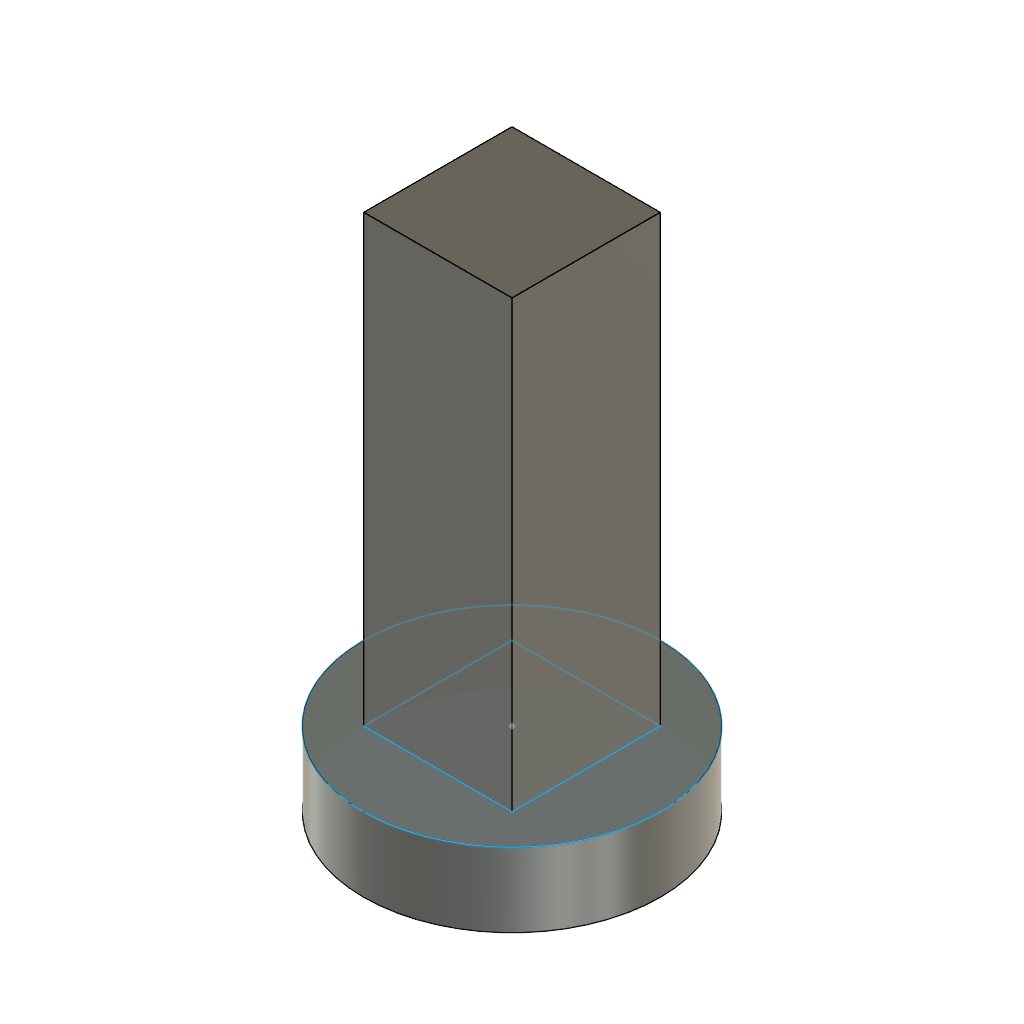
3d aiwa model (Autodesk Fusion 360 archive; units mm, degrees)
design "Screw"
part number: 2026-11-17-11-13-22-639
Autodesk Fusion 360 part; units mm, degrees
sketch "Sketch1" plane through (0, 0, 0) normal (0, 0, 1) x (1, 0, 0)
  circle A0 centre (-0.8105, -0.0035) radius 3
  line L0 (-2.3105, 1.4965) -> (0.6895, 1.4965)
  line L1 (0.6895, 1.4965) -> (0.6895, -1.5035)
  line L2 (0.6895, -1.5035) -> (-2.3105, -1.5035)
  line L3 (-2.3105, -1.5035) -> (-2.3105, 1.4965)
  dimension "d1" = 6
  dimension "d2" = 3
  dimension "d3" = 3
  dimension "d4" = 1.5
  dimension "d5" = 1.5
  constraint horizontal L0
  constraint vertical L1
  constraint horizontal L2
  constraint vertical L3
  measures "d1" diameter of A0
  measures "d2" distance of L0.start L0.end
  measures "d3" distance of L0.start L2.end
  measures "d4" distance of A0.centre L0
  measures "d5" distance of A0.centre L3
extrude "Extrude1" add sketch "Sketch1" against normal blind 1.5 contours A0 | L0 L1 L2 L3
extrude "Extrude2" add sketch "Sketch1" along normal blind 9 contours L0 L1 L2 L3
sketch "Sketch2" plane through (0, 0, -1.5) normal (0, 0, -1) x (1, 0, 0)
  circle A0 centre (-0.8105, 0.0035) radius 3
